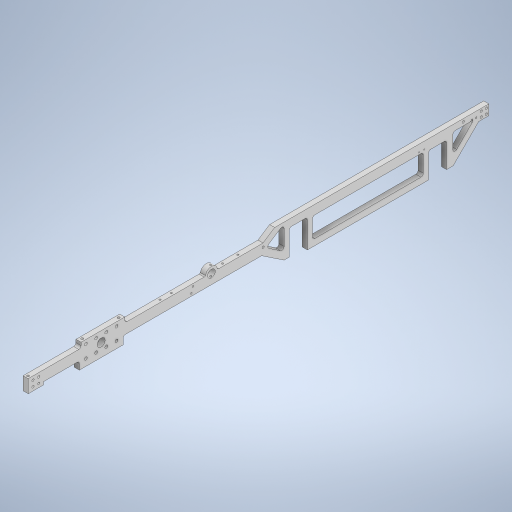
# Autodesk Inventor part: HUDSON 1-01-SIDE FRAME
Saved by Autodesk Inventor 2024.2 (Build 282272000, 272)
## iProperties
Created: 2024-09-28
Part Number: HUDSON 1-01-SIDE FRAME
Material: Generic
Document SubType Name: Modeling
Designer: Jimena Brenes
Density: 1 g/cm^3
Appearance: Default
Author: Jimena Brenes
Autodesk Inventor part; units mm, degrees
ref_plane "YZ Plane" through (0, 0, 0) normal (1, 0, 0) x (0, 1, 0)
ref_plane "XZ Plane" through (0, 0, 0) normal (0, 1, 0) x (-1, 0, 0)
ref_plane "XY Plane" through (0, 0, 0) normal (0, 0, 1) x (1, 0, 0)
sketch "Sketch1" plane through (0, 0, 0) normal (1, 0, 0) x (0, 1, 0)
  line L0 (-44.5, -450.4208) -> (-44.5, -459.4208)
  line L1 (-44.5, -459.4208) -> (0.5, -459.4208)
  line L2 (0.5, -459.4208) -> (0.5, -491.4208)
  line L3 (0.5, -491.4208) -> (-49.5, -491.4208)
  line L4 (-49.5, -491.4208) -> (-49.5, -704.4208)
  line L5 (-49.5, -704.4208) -> (-4.5, -704.4208)
  line L6 (-4.5, -704.4208) -> (-4.5, -736.4208)
  line L7 (-4.5, -736.4208) -> (-49.5, -736.4208)
  line L8 (-49.5, -736.4208) -> (-49.5, -747.9208)
  line L9 (-49.5, -747.9208) -> (-4.5, -792.9208)
  line L10 (-4.5, -792.9208) -> (-4.5, -810.9208)
  line L11 (-4.5, -810.9208) -> (13.5, -810.9208)
  line L12 (13.5, -810.9208) -> (13.5, -433.9208)
  line L13 (0, -170) -> (9, -170)
  line L14 (9, -93) -> (0, -93)
  line L15 (0, 0) -> (0, -93)
  line L16 (-44.5, -450.4208) -> (-18, -411)
  line L17 (-23, -27) -> (-18, -27)
  line L18 (-18, -27) -> (-18, -90)
  line L19 (-18, -90) -> (-32, -90)
  line L20 (-32, -90) -> (-32, -167)
  line L21 (-32, -167) -> (-18, -167)
  line L22 (-18, -411) -> (-18, -167)
  line L23 (9, -93) -> (9, -170)
  arc A0 (0, -333.3808) -> (0, -311.4719) centre (-1, -322.4263) ccw
  circle A1 centre (-1, -322.4263) radius 6.75
  line L24 (-23, -27) -> (-23, 0)
  line L25 (-23, 0) -> (0, 0)
  line L26 (0, -413.4208) -> (13.5, -433.9208)
  line L27 (0, -170) -> (0, -311.4719)
  line L28 (0, -333.3808) -> (0, -413.4208)
  dimension "d0" = 93
  dimension "d4" = 377
  dimension "d5" = 11.5
  dimension "d6" = 18
  dimension "d8" = 32
  dimension "d9" = 213
  dimension "d10" = 32
  dimension "d11" = 9
  dimension "d15" = 47.5
  dimension "d22" = 9
  dimension "d28" = 5
  dimension "d29" = 14
  dimension "d32" = 9
  dimension "d33" = 26.5
  dimension "d34" = 45
  dimension "d35" = 13
  dimension "d36" = 45
  dimension "d37" = 18
  dimension "d39" = 77
  dimension "d40" = 45
  dimension "d42" = 13.5
  dimension "d43" = 11
  dimension "d46" = 63
  dimension "d48" = 77
  dimension "d49" = 14
  dimension "d50" = 244
  dimension "d52" = 17
  dimension "d55" = 23
  dimension "d56" = 27
  dimension "d151" = 20.5
  constraints: 58 end point, 12 perpendicular, 8 vertical, 3 point on line, 2 centre point, 2 coincident, 2 horizontal, 2 point on circle, 1 parallel
  measures "d0" distance of L15.start L14.end
  measures "d4" distance of L11.end L12.end
  measures "d5" distance of L7.end L8.end
  measures "d6" distance of L9.end L10.end
  measures "d8" distance of L5.end L6.end
  measures "d9" distance of L3.end L4.end
  measures "d10" distance of L1.end L2.end
  measures "d11" distance of L0.start L0.end
  measures "d15" distance of L16.end L0.start
  measures "d22" distance of L14.start L14.end
  measures "d28" distance of L17.start L17.end
  measures "d29" distance of L18.end L19.end
  measures "d32" distance of L13.start L13.end
  measures "d33" distance between parallel lines of L22 L0
  measures "d34" distance of L0.end L1.end
  measures "d35" distance between parallel lines of L12 L2
  measures "d36" distance of L4.end L5.end
  measures "d37" distance of L10.end L11.end
  measures "d39" distance of L14.start L13.end
  measures "d40" distance of L6.end L7.end
  measures "d42" diameter of A1
  measures "d43" radius of A0
  measures "d46" distance of L17.end L18.end
  measures "d48" distance of L19.end L20.end
  measures "d49" distance of L20.end L21.end
  measures "d50" distance of L16.end L21.end
  measures "d52" distance from line of L22 A1.centre
  measures "d55" distance of L24.end L15.start
  measures "d56" distance of L17.start L24.end
  measures "d151" vertical distance of L12.end L26.start
extrude "Extrusion1" add sketch "Sketch1" along normal blind 9
sketch "Sketch2" plane through (9, 0, 0) normal (1, 0, 0) x (0, 0, -1)
  line L0 (0, -23) -> (27, -23) projected
  line L1 (8.5, -6.5) -> (18.5, -6.5) construction
  line L2 (18.5, -6.5) -> (18.5, -16.5) construction
  line L3 (18.5, -16.5) -> (8.5, -16.5) construction
  line L4 (8.5, -16.5) -> (8.5, -6.5) construction
  circle A0 centre (8.5, -6.5) radius 2
  circle A1 centre (18.5, -6.5) radius 2
  circle A2 centre (18.5, -16.5) radius 2
  circle A3 centre (8.5, -16.5) radius 2
  line L5 (797.4208, 9) -> (806.4208, 9) construction
  line L6 (806.4208, 9) -> (806.4208, 0) construction
  line L7 (806.4208, 0) -> (797.4208, 0) construction
  line L8 (797.4208, 0) -> (797.4208, 9) construction
  circle A4 centre (806.4208, 9) radius 2
  circle A5 centre (797.4208, 9) radius 2
  circle A6 centre (797.4208, 0) radius 2
  circle A7 centre (806.4208, 0) radius 2
  line L9 (792.9208, -4.5) -> (810.9208, -4.5) projected
  line L10 (810.9208, -4.5) -> (810.9208, 13.5) projected
  circle A8 centre (788.4208, 3.5) radius 1.5
  circle A9 centre (781.4208, 3.5) radius 1.5
  line L11 (810.9208, 13.5) -> (433.9208, 13.5) projected
  line L12 (0, 0) -> (0, -23) projected
  line L13 (93, 0) -> (0, 0) projected
  line L14 (155.5, -20) -> (101.5, -20) construction
  line L15 (101.5, -20) -> (101.5, 2) construction
  line L16 (101.5, 2) -> (155.5, 2) construction
  line L17 (155.5, 2) -> (155.5, -20) construction
  line L18 (101.5, -20) -> (155.5, 2) construction
  circle A10 centre (101.5, 2) radius 2.5
  circle A11 centre (119.5, 2) radius 2.5
  circle A12 centre (137.5, 2) radius 2.5
  circle A13 centre (155.5, 2) radius 2.5
  circle A14 centre (155.5, -20) radius 2.5
  circle A15 centre (137.5, -20) radius 2.5
  circle A16 centre (119.5, -20) radius 2.5
  circle A17 centre (101.5, -20) radius 2.5
  line L19 (170, 9) -> (93, 9) projected
  line L20 (90, -18) -> (90, -32) projected
  line L21 (167, -32) -> (167, -18) projected
  line L22 (90, -32) -> (167, -32) projected
  circle A18 centre (128.5, -9) radius 7
  circle A19 centre (290, -4.5) radius 1.5
  circle A20 centre (287, -13.5) radius 1.5
  line L23 (167, -18) -> (411, -18) projected
  line L24 (170, 0) -> (170, 9) projected
  dimension "d63" = 4
  dimension "d64" = 4
  dimension "d65" = 4
  dimension "d66" = 4
  dimension "d67" = 4
  dimension "d68" = 4
  dimension "d69" = 4
  dimension "d70" = 4
  dimension "d71" = 4.5
  dimension "d72" = 4.5
  dimension "d73" = 9
  dimension "d74" = 9
  dimension "d75" = 3
  dimension "d76" = 3
  dimension "d77" = 9
  dimension "d78" = 7
  dimension "d80" = 8
  dimension "d81" = 8
  dimension "d82" = 10
  dimension "d83" = 8.5
  dimension "d84" = 6.5
  dimension "d85" = 10
  dimension "d86" = 5
  dimension "d87" = 5
  dimension "d88" = 5
  dimension "d89" = 5
  dimension "d90" = 5
  dimension "d91" = 5
  dimension "d92" = 5
  dimension "d93" = 5
  dimension "d95" = 7
  dimension "d96" = 11.5
  dimension "d97" = 18
  dimension "d98" = 18
  dimension "d99" = 18
  dimension "d100" = 11.5
  dimension "d102" = 41
  dimension "d105" = 22
  dimension "d106" = 18
  dimension "d107" = 18
  dimension "d108" = 14
  dimension "d111" = 3
  dimension "d112" = 3
  dimension "d113" = 4.5
  dimension "d114" = 9
  dimension "d115" = 120
  dimension "d116" = 120
  constraints: 26 end point, 21 centre point, 13 coincident, 6 parallel, 4 point on line, 3 horizontal, 3 perpendicular, 1 midpoint
  measures "d63" diameter of A0
  measures "d64" diameter of A1
  measures "d65" diameter of A2
  measures "d66" diameter of A3
  measures "d67" diameter of A4
  measures "d68" diameter of A5
  measures "d69" diameter of A6
  measures "d70" diameter of A7
  measures "d71" distance from line of L9 L6.end
  measures "d72" distance from line of L10 L6.end
  measures "d73" distance of L7.end L6.end
  measures "d74" distance of L6.end L5.end
  measures "d75" diameter of A8
  measures "d76" diameter of A9
  measures "d77" horizontal distance of L7.end A8.centre
  measures "d78" distance of A9.centre A8.centre
  measures "d80" distance from line of L9 A8.centre
  measures "d81" distance from line of L9 A9.centre
  measures "d82" distance of L3.end L1.start
  measures "d83" distance from line of L12 L3.end
  measures "d84" distance from line of L13 L1.start
  measures "d85" distance of L2.end L3.end
  measures "d86" diameter of A10
  measures "d87" diameter of A11
  measures "d88" diameter of A12
  measures "d89" diameter of A13
  measures "d90" diameter of A14
  measures "d91" diameter of A15
  measures "d92" diameter of A16
  measures "d93" diameter of A17
  measures "d95" distance from line of L19 L15.end
  measures "d96" distance from line of L20 L14.end
  measures "d97" distance of A16.centre A17.centre
  measures "d98" distance of A15.centre A16.centre
  measures "d99" distance of L14.start A15.centre
  measures "d100" distance from line of L21 A14.centre
  measures "d102" distance between parallel lines of L22 L19
  measures "d105" distance of A17.centre L15.end
  measures "d106" distance of A11.centre L15.end
  measures "d107" distance of A11.centre A12.centre
  measures "d108" diameter of A18
  measures "d111" diameter of A19
  measures "d112" diameter of A20
  measures "d113" distance from line of L23 A20.centre
  measures "d114" vertical distance of A20.centre A19.centre
  measures "d115" distance from line of L21 A20.centre
  measures "d116" distance from line of L24 A19.centre
fillet "Fillet1" radius 4 4 edges at (4.5, 0, -170) (4.5, -18, -167) (4.5, -18, -90) (4.5, 0, -93)
hole "Hole1" at (9, -6.5, -8.5) at (9, -16.5, -8.5) at (9, -16.5, -18.5) at (9, -6.5, -18.5) at (9, 9, -806.4208) at (9, 0, -806.4208) at (9, 0, -797.4208) at (9, 9, -797.4208) direction (-1, 0, 0) diameter 4 end through all
hole "Hole2" at (9, 3.5, -788.4208) at (9, 3.5, -781.4208) at (9, -4.5, -290) at (9, -13.5, -287) direction (-1, 0, 0) diameter 3 end through all
hole "Hole3" at (9, 2, -101.5) at (9, -20, -101.5) at (9, 2, -119.5) at (9, -20, -119.5) at (9, -20, -137.5) at (9, 2, -137.5) at (9, 2, -155.5) at (9, -20, -155.5) direction (-1, 0, 0) diameter 5 end through all
hole "Hole4" at (9, -9, -128.5) direction (-1, 0, 0) diameter 14 end through all
sketch "Sketch3" plane through (9, 0, 0) normal (1, 0, 0) x (0, 0, -1)
  line L0 (411, -18) -> (450.4208, -44.5) projected
  line L1 (459.4208, -44.5) -> (459.4208, 0.5) projected
  line L2 (433.9208, 13.5) -> (413.4208, 0) projected
  line L3 (450.4208, -23.7369) -> (450.4208, 3.7713)
  line L4 (444.2208, 7.112) -> (423.55, -6.5005)
  line L5 (423.5184, -13.1609) -> (444.1892, -27.0565)
  arc A0 (423.55, -6.5005) -> (423.5184, -13.1609) centre (425.75, -9.8412) ccw
  arc A1 (450.4208, 3.7713) -> (444.2208, 7.112) centre (446.4208, 3.7713) ccw
  arc A2 (444.1892, -27.0565) -> (450.4208, -23.7369) centre (446.4208, -23.7369) ccw
  line L6 (500.4208, -2.5) -> (695.4208, -2.5)
  line L7 (695.4208, -2.5) -> (695.4208, -38.5)
  line L8 (695.4208, -38.5) -> (500.4208, -38.5)
  line L9 (500.4208, -38.5) -> (500.4208, -2.5)
  line L10 (491.4208, -49.5) -> (704.4208, -49.5) projected
  line L11 (491.4208, 0.5) -> (491.4208, -49.5) projected
  line L12 (704.4208, -49.5) -> (704.4208, -4.5) projected
  circle A3 centre (413.4263, -6.5) radius 2
  line L13 (413.4208, 0) -> (333.3808, 0) projected
  circle A4 centre (322.4263, -1) radius 6.75 projected
  line L14 (747.4208, 2.5) -> (747.4208, -34.4437)
  line L15 (747.4208, -34.4437) -> (784.3645, 2.5)
  line L16 (784.3645, 2.5) -> (747.4208, 2.5)
  line L17 (736.4208, -4.5) -> (736.4208, -49.5) projected
  line L18 (810.9208, 13.5) -> (433.9208, 13.5) projected
  line L19 (747.9208, -49.5) -> (792.9208, -4.5) projected
  circle A5 centre (765.9208, 8.5) radius 2
  line L20 (687.9208, 1) -> (696.9208, 1) construction
  circle A6 centre (696.9208, 1) radius 1
  circle A7 centre (687.9208, 1) radius 1
  line L21 (704.4208, -4.5) -> (736.4208, -4.5) projected
  circle A8 centre (779.536, 0.5) radius 2
  point P0 (0, 0)
  point P1 (423.6708, 6.75)
  dimension "d154" = 9
  dimension "d155" = 11
  dimension "d157" = 8
  dimension "d158" = 8
  dimension "d159" = 8
  dimension "d160" = 11
  dimension "d161" = 36
  dimension "d162" = 11
  dimension "d163" = 9
  dimension "d164" = 9
  dimension "d165" = 4
  dimension "d166" = 6.5
  dimension "d167" = 91
  dimension "d168" = 11
  dimension "d169" = 11
  dimension "d170" = 11
  dimension "d171" = 4
  dimension "d172" = 18.5
  dimension "d173" = 5
  dimension "d174" = 2
  dimension "d175" = 2
  dimension "d176" = 9
  dimension "d177" = 5.5
  dimension "d178" = 187.5
  dimension "d204" = 4
  constraints: 22 end point, 8 centre point, 8 parallel, 8 tangent, 6 point on circle, 2 coincident, 2 horizontal, 2 perpendicular, 2 vertical, 1 midpoint
  measures "d154" distance between parallel lines of L1 L3
  measures "d155" distance between parallel lines of L0 L5
  measures "d157" diameter of A0
  measures "d158" diameter of A1
  measures "d159" diameter of A2
  measures "d160" distance from line of point (423.671, 6.75) L4
  measures "d161" distance between parallel lines of L8 L6
  measures "d162" distance between parallel lines of L10 L8
  measures "d163" distance between parallel lines of L11 L9
  measures "d164" distance between parallel lines of L12 L7
  measures "d165" diameter of A3
  measures "d166" distance from line of L13 A3.centre
  measures "d167" horizontal distance of A4.centre A3.centre
  measures "d168" distance between parallel lines of L17 L14
  measures "d169" distance between parallel lines of L19 L15
  measures "d170" distance between parallel lines of L18 L16
  measures "d171" diameter of A5
  measures "d172" distance from line of L14 A5.centre
  measures "d173" distance from line of L18 A5.centre
  measures "d174" diameter of A6
  measures "d175" diameter of A7
  measures "d176" distance of L20.end L20.start
  measures "d177" distance from line of L21 L20.end
  measures "d178" distance from line of L9 A7.centre
  measures "d204" diameter of A8
extrude "Extrusion2" cut sketch "Sketch3" against normal through all contours A2 L5 A0 L4 A1 L3 | L6 L7 L8 L9 | L16 A8 L15 L14 | L16 L15 A8 | A8
fillet "Fillet2" radius 4 11 edges at (4.5, -2.5, -695.4208) (4.5, -38.5, -695.4208) (4.5, -38.5, -500.4208) (4.5, -2.5, -500.4208) (4.5, 2.5, -747.4208) (4.5, -34.4437, -747.4208) (4.5, 2.5, -784.3645) (4.5, -4.5, -736.4208) (4.5, -4.5, -704.4208) (4.5, 0.5, -491.4208) (4.5, 0.5, -459.4208)
hole "Hole5" at (9, -6.5, -413.4263) direction (-1, 0, 0) diameter 4 end through all
hole "Hole6" at (9, 1, -687.9208) at (9, 1, -696.9208) direction (-1, 0, 0) diameter 2 end through all
hole "Hole7" at (9, 8.5, -765.9208) direction (-1, 0, 0) diameter 4 end through all
fillet "Fillet3" radius 2 2 edges at (4.5, 0, -311.4719) (4.5, 0, -333.3808)
sketch "Sketch4" plane through (0, 0, 0) normal (0, 1, 0) x (1, 0, 0)
  circle A0 centre (4.5, 4) radius 2
  line L0 (9, 89) -> (9, 0) projected
  line L1 (0, 0) -> (9, 0) projected
  dimension "d205" = 4
  dimension "d206" = 4.5
  dimension "d207" = 4
  constraints: 1 centre point
  measures "d205" diameter of A0
  measures "d206" distance from line of L0 A0.centre
  measures "d207" distance from line of L1 A0.centre
hole "Hole8" at (4.5, 0, -4) direction (0, -1, 0) diameter 4 end through all
sketch "Sketch5" plane through (0, 9, -93) normal (0, 1, 0) x (1, 0, 0)
  circle A0 centre (4.5, 6.5) radius 2
  circle A1 centre (4.5, 70.5) radius 2
  circle A2 centre (4.5, -89) radius 2 projected
  circle A3 centre (4.5, -89) radius 2 projected
  line L0 (0, -4) -> (9, -4) projected
  line L1 (0, -4) -> (0, -93) projected
  line L2 (0, -93) -> (9, -93) projected
  line L3 (9, -4) -> (9, -93) projected
  line L4 (9, 77) -> (9, 0) projected
  circle A4 centre (4.5, 143.5) radius 1.5
  line L5 (9, 216.7772) -> (9, 81) projected
  circle A5 centre (4.5, 163.5) radius 1.5
  circle A6 centre (6, 231) radius 1.5
  circle A7 centre (4.5, 253.5) radius 1.5
  circle A8 centre (4.5, 280.5) radius 1.5
  line L6 (9, 320.4208) -> (9, 242.0754) projected
  dimension "d215" = 4
  dimension "d216" = 4
  dimension "d217" = 95.5
  dimension "d218" = 64
  dimension "d219" = 4.5
  dimension "d220" = 4.5
  dimension "d221" = 3
  dimension "d222" = 73
  dimension "d223" = 4.5
  dimension "d224" = 3
  dimension "d225" = 20
  dimension "d226" = 4.5
  dimension "d227" = 3
  dimension "d228" = 67.5
  dimension "d229" = 3
  dimension "d230" = 22.5
  dimension "d231" = 3
  dimension "d232" = 4.5
  dimension "d233" = 27
  dimension "d234" = 4.5
  constraints: 7 centre point
  measures "d215" diameter of A0
  measures "d216" diameter of A1
  measures "d217" distance of A2.centre A0.centre
  measures "d218" distance of A0.centre A1.centre
  measures "d219" distance from line of L4 A0.centre
  measures "d220" distance from line of L4 A1.centre
  measures "d221" diameter of A4
  measures "d222" distance of A1.centre A4.centre
  measures "d223" distance from line of L5 A4.centre
  measures "d224" diameter of A5
  measures "d225" distance of A5.centre A4.centre
  measures "d226" distance from line of L5 A5.centre
  measures "d227" diameter of A6
  measures "d228" vertical distance of A6.centre A5.centre
  measures "d229" diameter of A7
  measures "d230" vertical distance of A6.centre A7.centre
  measures "d231" diameter of A8
  measures "d232" distance from line of L6 A7.centre
  measures "d233" distance of A8.centre A7.centre
  measures "d234" distance from line of L6 A8.centre
hole "Hole9" at (4.5, 9, -99.5) at (4.5, 9, -163.5) direction (0, -1, 0) diameter 4 end through all
hole "Hole10" at (4.5, 9, -236.5) at (4.5, 9, -256.5) at (6, 9, -324) at (4.5, 9, -346.5) at (4.5, 9, -373.5) direction (0, -1, 0) diameter 3 end through all both
body "Solid1"
